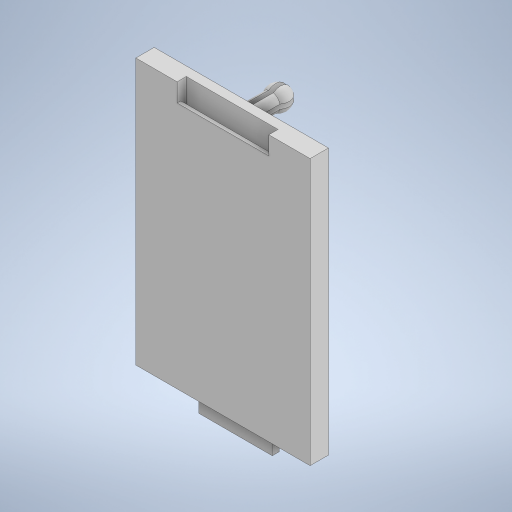
# Autodesk Inventor part: trappe
Saved by Autodesk Inventor 2024.2 (Build 282272000, 272)
## iProperties
Created: 2024-05-24
Part Number: trappe
Material: Générique
Document SubType Name: Modeling
Designer: michgae
Density: 1 g/cm^3
Appearance: Par défaut
Author: michgae
Autodesk Inventor part; units mm, degrees
ref_plane "YZ Plane" through (0, 0, 0) normal (1, 0, 0) x (0, 1, 0)
ref_plane "XZ Plane" through (0, 0, 0) normal (0, 1, 0) x (-1, 0, 0)
ref_plane "XY Plane" through (0, 0, 0) normal (0, 0, 1) x (1, 0, 0)
sketch "Esquisse1" plane through (0, 0, 0) normal (0, 0, 1) x (1, 0, 0)
  line L0 (-9.5, 14.5) -> (9.5, 14.5)
  line L1 (9.5, 14.5) -> (9.5, -14.5)
  line L2 (9.5, -14.5) -> (-9.5, -14.5)
  line L3 (-9.5, -14.5) -> (-9.5, 14.5)
  line L4 (-13.3, 0) -> (13.3, 0) projected
  line L5 (0, -20.3) -> (0, 20.3) projected
  circle A0 centre (0, 12.5) radius 1
  point P0 (0, 0)
  dimension "d0" = 19
  dimension "d1" = 29
  dimension "d2" = 2
  dimension "d3" = 2
  constraints: 8 end point, 2 parallel, 1 centre point, 1 horizontal, 1 perpendicular, 1 point on line, 2 other
  measures "d0" distance of L0.start L0.end
  measures "d1" distance of L0.end L1.end
  measures "d2" diameter of A0
  measures "d3" distance from line of L0 A0.centre
extrude "Extrusion1" add sketch "Esquisse1" along normal blind 2 contours L0 L5 A0 L4 L3 | L0 L1 L4 L5 A0 | L4 L5 L2 L3 | L4 L1 L2 L5
sketch "Esquisse2" plane through (0, 0, 0) normal (0, 0, -1) x (-1, 0, 0)
  line L0 (-4, -12) -> (4, -12)
  line L1 (4, -12) -> (4, -17)
  line L2 (4, -17) -> (-4, -17)
  line L3 (-4, -17) -> (-4, -12)
  line L4 (0, -23.3) -> (0, 20.8) projected
  line L5 (9.5, -14.5) -> (-9.5, -14.5) projected
  point P0 (0, 0)
  dimension "d6" = 8
  dimension "d7" = 5
  dimension "d8" = 2.5
  constraints: 8 end point, 2 parallel, 1 horizontal, 1 perpendicular, 1 other
  measures "d6" distance of L1.end L2.end
  measures "d7" distance of L0.end L1.end
  measures "d8" distance between parallel lines of L5 L0
extrude "Extrusion2" add sketch "Esquisse2" along normal mid plane 1.25
chamfer "Chanfrein1" distance 0.5 angle 45 3 edges at (0, -12, -0.625) (4, -14.5, -0.625) (-4, -14.5, -0.625)
extrude "Extrusion3" add sketch "Esquisse1" against normal blind 4 contours A0 L5 | L5 A0
sketch "Esquisse3" plane through (0, 12.5, -4) normal (0, 0, -1) x (-1, 0, 0)
  arc A0 (0, -1.25) -> (0, 1.25) centre (0, 0) ccw
  line L0 (0, 1.25) -> (0, -1.25)
  line L1 (0.25, 1.3454) -> (0.25, -1.2696)
  line L2 (-0.25, 1.3454) -> (-0.25, -1.2696)
  line L3 (-0.25, 1.3454) -> (0.25, 1.3454)
  line L4 (0.25, -1.2696) -> (-0.25, -1.2696)
  line L5 (-0.9682, 0.25) -> (0.9682, 0.25)
  circle A1 centre (0, 0) radius 1 projected
  line L6 (-0.9015, -0.25) -> (1.035, -0.25)
  circle A2 centre (0, 0) radius 1 projected
  line L7 (-0.9682, 0.25) -> (-1.0579, 0.25)
  line L8 (-1.0579, -0.25) -> (-0.9015, -0.25)
  line L9 (1.035, 0.25) -> (0.9682, 0.25)
  line L10 (1.035, 0.25) -> (1.2927, 0.25)
  line L11 (1.2927, 0.25) -> (1.2927, -0.25)
  line L12 (1.2927, -0.25) -> (1.035, -0.25)
  line L13 (-1.0579, 0.25) -> (-1.4678, 0.25)
  line L14 (-1.4678, 0.25) -> (-1.4678, -0.25)
  line L15 (-1.4678, -0.25) -> (-1.0579, -0.25)
  point P0 (0, -12.5)
  point P1 (0, 0)
  point P2 (0.25, 0.25)
  point P3 (-0.25, 0.25)
  point P4 (-0.25, -0.25)
  point P5 (0.25, -0.25)
  point P6 (0, 1.2247)
  point P7 (0, -1.2247)
  point P8 (1.2247, 0.25)
  point P9 (0.25, 1.2247)
  point P10 (1.2247, -0.25)
  point P11 (0.25, -1.2247)
  point P12 (0, -0.25)
  point P13 (0, 0.25)
  dimension "d16" = 1.25
  dimension "d17" = 0
  dimension "d18" = 0
  dimension "d19" = 13.75
  dimension "d21" = 0.25
  dimension "d22" = 0.25
  dimension "d56" = 1.0427
  dimension "d57" = 2.7604
  dimension "d58" = 0.5
  dimension "d59" = 1.0954
  dimension "d60" = 1.5196
  dimension "d61" = 0.2577
  dimension "d62" = 0.2577
  dimension "d63" = 1.0427
  dimension "d64" = 1.0427
  dimension "d65" = 1.0954
  dimension "d66" = 1.0427
  dimension "d67" = 0.5
  dimension "d68" = 1.0427
  dimension "d69" = 0
  dimension "d70" = 1.2927
  dimension "d71" = 0.9747
  dimension "d72" = 1.2927
  dimension "d73" = 1.4747
  dimension "d74" = 1.5427
  dimension "d75" = 0
  dimension "d76" = 1.5427
  dimension "d77" = 0.5
  dimension "d78" = 2.3506
  dimension "d79" = 2.3506
  constraints: 32 end point, 6 horizontal, 5 parallel, 4 perpendicular, 2 point on circle, 2 point on line, 2 vertical, 1 centre point, 1 midpoint, 5 other
  measures "d16" radius of A0
  measures "d17" distance from line of point (0, -12.5) L0
  measures "d18" distance from line of A0.centre L0
  measures "d19" distance of point (0, -12.5) L0.start
  measures "d21" distance between parallel lines of L0 L1
  measures "d22" distance from line of point (0, 0) L5
  measures "d56" distance between parallel lines of L1 L11
  measures "d57" distance between parallel lines of L11 L14
  measures "d58" distance between parallel lines of L15 L5
  measures "d59" distance between parallel lines of L3 L10
  measures "d60" distance between parallel lines of L4 L5
  measures "d61" distance from line of L9.start L11
  measures "d62" distance from line of L6.end L11
  measures "d63" distance from line of L3.end L11
  measures "d64" distance from line of point (0.25, 1.345) L11
  measures "d65" distance from line of point (0.25, 1.345) L5
  measures "d66" distance from line of point (0.25, 0.25) L11
  measures "d67" distance from line of point (0.25, 0.25) L12
  measures "d68" distance from line of point (0.25, -0.25) L11
  measures "d69" distance from line of point (0.25, -0.25) L12
  measures "d70" distance from line of point (0, 1.225) L11
  measures "d71" distance from line of point (0, 1.225) L5
  measures "d72" distance from line of point (0, -1.225) L11
  measures "d73" distance from line of point (0, -1.225) L5
  measures "d74" distance from line of point (-0.25, 0.25) L11
  measures "d75" distance from line of point (-0.25, 0.25) L5
  measures "d76" distance from line of point (-0.25, -0.25) L11
  measures "d77" distance from line of point (-0.25, -0.25) L5
  measures "d78" distance from line of L7.end L11
  measures "d79" distance from line of L8.start L11
revolve "Révolution1" add sketch "Esquisse3" angle 360 about axis through (0, 13.75, -4) along (0, -1, 0) contours L0 A1 L1 A0 | L1 A1 L6 L12 A0 | L0 L6 L1 A1 | L12 L6 A1 L9 L10 A0 | L1 L6 A1 | L0 L5 L1 L6 | L10 L9 A1 L1 A0 | L1 L5 A1 L6 | L0 A1 L1 L5 | L1 A1 L0 A0 | L1 A1 L5
extrude "Extrusion6" cut sketch "Esquisse3" along normal blind 4 and the other way blind 3 contours L0 A1 L1 A0 | A0 L1 L4 L2 A1 L0 | A1 L2 L6 L0 | L0 L6 L1 A1 | L12 L6 A1 L9 L10 A0 | A0 L10 L11 L12 | L6 L2 L5 L0 | L0 L5 L1 L6 | L1 L5 A1 L6 | L5 L2 A1 L0 | L0 A1 L1 L5 | L6 L8 A1 L5 L2 | L8 L15 L14 L13 L7 A1 | L1 A1 L0 A0 | A0 L0 A1 L2 L3 L1
sketch "Esquisse4" plane through (0, 12.5, 0) normal (0, 0, 1) x (1, 0, 0)
  circle A0 centre (0, 0) radius 1
  point P0 (0, -12.5)
  constraints: 1 centre point
extrude "Extrusion7" add sketch "Esquisse4" along normal blind 2
sketch "Esquisse5" plane through (-9.5, 14.5, 0) normal (0, 1, 0) x (1, 0, 0)
  line L0 (19, -2) -> (0, -2) projected
  line L1 (14.5, -2) -> (4.5, -2)
  line L2 (4.5, -2) -> (4.5, -1)
  line L3 (4.5, -1) -> (14.5, -1)
  line L4 (14.5, -1) -> (14.5, -2)
  line L5 (19, 0) -> (19, -2) projected
  point P0 (9.5, 0)
  point P1 (14.5, -1.5)
  dimension "d86" = 10
  dimension "d87" = 4.5
  dimension "d88" = 1
  constraints: 8 end point, 2 parallel, 1 horizontal, 1 midpoint, 1 perpendicular, 1 point on line
  measures "d86" distance of L2.end L3.end
  measures "d87" distance from line of L5 point (14.5, -1.5)
  measures "d88" distance of L3.end L1.start
extrude "Extrusion8" cut sketch "Esquisse5" against normal blind 2
sketch "Esquisse6" plane through (-9.5, 12.5, 0) normal (0, 1, 0) x (1, 0, 0)
  line L0 (4.5, -2) -> (4.5, -1) projected
  line L1 (14.5, -1) -> (14.5, -2) projected
  line L2 (4.5, -1) -> (14.5, -1)
  line L3 (14.5, -1) -> (14.5, -1.6)
  line L4 (14.5, -1.6) -> (4.5, -1.6)
  line L5 (4.5, -1.6) -> (4.5, -1)
  point P0 (9.5, 0)
  dimension "d91" = 0.6
  constraints: 8 end point, 2 parallel, 1 horizontal, 1 perpendicular, 1 point on line
  measures "d91" distance of L2.end L3.end
extrude "Extrusion9" cut sketch "Esquisse6" against normal blind 2
